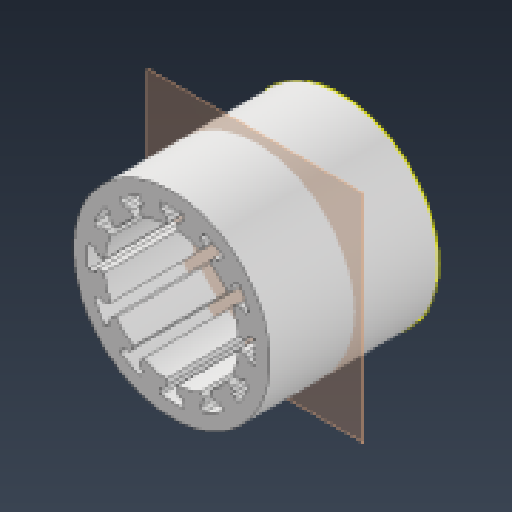
# Autodesk Inventor part: СИСЬКА
Saved by Autodesk Inventor 2026 (Build 300175000, 175)
## iProperties
Created: 2025-10-03
Part Number: СИСЬКА
Material: Типовые
Document SubType Name: Modeling
Designer: Phantom
Density: 1 g/cm^3
Appearance: По умолчанию
Author: Phantom
Autodesk Inventor part; units mm, degrees
ref_plane "YZ Plane" through (0, 0, 0) normal (1, 0, 0) x (0, 1, 0)
ref_plane "XZ Plane" through (0, 0, 0) normal (0, 1, 0) x (-1, 0, 0)
ref_plane "XY Plane" through (0, 0, 0) normal (0, 0, 1) x (1, 0, 0)
sketch "Эскиз1" plane through (0, 0, 0) normal (0, 0, 1) x (1, 0, 0)
  line L0 (-8.756, -8.6711) -> (-8.756, 8.8289)
  line L1 (-8.756, 8.8289) -> (8.744, 8.8289)
  line L2 (8.744, 8.8289) -> (8.744, -8.6711)
  line L3 (8.744, -8.6711) -> (-8.756, -8.6711)
  arc A0 (13.9306, 22.0467) -> (13.3924, 24.6651) centre (12.555, 23.1285) ccw
  line L4 (9.474, 16.3796) -> (13.9306, 22.0467)
  arc A1 (7.3589, 15.8753) -> (9.474, 16.3796) centre (8.0984, 17.4614) ccw
  arc A2 (7.3589, 15.8753) -> (5.5646, 16.5937) centre (-0.006, 0.0789) ccw
  arc A3 (4.3818, 18.4182) -> (5.5646, 16.5937) centre (6.1239, 18.2519) ccw
  line L5 (5.0671, 25.5951) -> (4.3818, 18.4182)
  arc A4 (7.2635, 27.1187) -> (5.0671, 25.5951) centre (6.8092, 25.4288) ccw
  arc A5 (7.2635, 27.1187) -> (-2.0268, 28.0059) centre (-0.006, 0.0789) ccw
  arc A6 (-0.1585, 26.0941) -> (-2.0268, 28.0059) centre (-1.9005, 26.2604) ccw
  line L6 (-0.8438, 18.9172) -> (-0.1585, 26.0941)
  arc A7 (-2.3505, 17.3495) -> (-0.8438, 18.9172) centre (-2.5859, 19.0836) ccw
  arc A8 (-2.3505, 17.3495) -> (-4.2483, 16.9837) centre (-0.006, 0.0789) ccw
  arc A9 (-6.2297, 17.8792) -> (-4.2483, 16.9837) centre (-4.6743, 18.6811) ccw
  line L7 (-9.5333, 24.2872) -> (-6.2297, 17.8792)
  arc A10 (-8.5093, 26.7565) -> (-9.5333, 24.2872) centre (-7.9779, 25.0891) ccw
  arc A11 (-8.5093, 26.7565) -> (-16.8045, 22.48) centre (-0.006, 0.0789) ccw
  arc A12 (-14.1991, 21.8818) -> (-16.8045, 22.48) centre (-15.7546, 21.0799) ccw
  line L8 (-10.8956, 15.4738) -> (-14.1991, 21.8818)
  arc A13 (-11.3155, 13.3403) -> (-10.8956, 15.4738) centre (-12.451, 14.6719) ccw
  arc A14 (-11.3155, 13.3403) -> (-12.7143, 12.0065) centre (-0.006, 0.0789) ccw
  arc A15 (-14.8653, 11.6886) -> (-12.7143, 12.0065) centre (-13.9903, 13.2042) ccw
  line L9 (-21.1089, 15.2934) -> (-14.8653, 11.6886)
  arc A16 (-21.5824, 17.9243) -> (-21.1089, 15.2934) centre (-20.2339, 16.8089) ccw
  arc A17 (-21.5824, 17.9243) -> (-26.2488, 9.842) centre (-0.006, 0.0789) ccw
  arc A18 (-23.7336, 10.7473) -> (-26.2488, 9.842) centre (-24.6086, 9.2318) ccw
  line L10 (-17.49, 7.1425) -> (-23.7336, 10.7473)
  arc A19 (-16.6898, 5.1208) -> (-17.49, 7.1425) centre (-18.365, 5.627) ccw
  arc A20 (-16.6898, 5.1208) -> (-17.1455, 3.2424) centre (-0.006, 0.0789) ccw
  arc A21 (-18.7831, 1.8121) -> (-17.1455, 3.2424) centre (-18.8664, 3.5601) ccw
  line L11 (-25.9845, 1.469) -> (-18.7831, 1.8121)
  arc A22 (-27.8052, 3.4263) -> (-25.9845, 1.469) centre (-26.0677, 3.217) ccw
  arc A23 (-27.8052, 3.4263) -> (-27.3611, -5.8958) centre (-0.006, 0.0789) ccw
  arc A24 (-25.7347, -3.7744) -> (-27.3611, -5.8958) centre (-25.6514, -5.5224) ccw
  line L12 (-18.5334, -3.4313) -> (-25.7347, -3.7744)
  arc A25 (-16.7671, -4.6996) -> (-18.5334, -3.4313) centre (-18.4501, -5.1793) ccw
  arc A26 (-16.7671, -4.6996) -> (-16.135, -6.5261) centre (-0.006, 0.0789) ccw
  arc A27 (-16.7394, -8.6147) -> (-16.135, -6.5261) centre (-17.7545, -7.1892) ccw
  line L13 (-22.6121, -12.7967) -> (-16.7394, -8.6147)
  arc A28 (-25.2019, -12.1345) -> (-22.6121, -12.7967) centre (-23.6272, -11.3712) ccw
  arc A29 (-25.2019, -12.1345) -> (-19.7884, -19.7366) centre (-0.006, 0.0789) ccw
  arc A30 (-19.5671, -17.0727) -> (-19.7884, -19.7366) centre (-18.552, -18.4982) ccw
  line L14 (-13.6944, -12.8907) -> (-19.5671, -17.0727)
  arc A31 (-11.523, -13.0028) -> (-13.6944, -12.8907) centre (-12.6793, -14.3162) ccw
  arc A32 (-11.523, -13.0028) -> (-10.0037, -14.1975) centre (-0.006, 0.0789) ccw
  arc A33 (-9.3829, -16.2814) -> (-10.0037, -14.1975) centre (-11.0075, -15.631) ccw
  line L15 (-12.0624, -22.9745) -> (-9.3829, -16.2814)
  arc A34 (-14.5991, -23.8176) -> (-12.0624, -22.9745) centre (-13.687, -22.3241) ccw
  arc A35 (-14.5991, -23.8176) -> (-5.935, -27.2862) centre (-0.006, 0.0789) ccw
  arc A36 (-7.189, -24.9255) -> (-5.935, -27.2862) centre (-5.5644, -25.5759) ccw
  line L16 (-4.5095, -18.2324) -> (-7.189, -24.9255)
  arc A37 (-2.6222, -17.1526) -> (-4.5095, -18.2324) centre (-2.8849, -18.8828) ccw
  arc A38 (-2.6222, -17.1526) -> (-0.6982, -17.3363) centre (-0.006, 0.0789) ccw
  arc A39 (0.9507, -18.7538) -> (-0.6982, -17.3363) centre (-0.7677, -19.085) ccw
  line L17 (2.3151, -25.833) -> (0.9507, -18.7538)
  arc A40 (0.6369, -27.9137) -> (2.3151, -25.833) centre (0.5967, -26.1642) ccw
  arc A41 (0.6369, -27.9137) -> (9.8009, -26.1475) centre (-0.006, 0.0789) ccw
  arc A42 (7.4696, -24.8396) -> (9.8009, -26.1475) centre (9.188, -24.5084) ccw
  line L18 (6.1065, -17.7672) -> (7.4696, -24.8396)
  arc A43 (7.1038, -15.8414) -> (6.1065, -17.7672) centre (7.8249, -17.436) ccw
  arc A44 (7.1038, -15.8414) -> (8.8253, -14.9478) centre (-0.2779, 0.4827) ccw
  arc A45 (10.981, -15.2474) -> (8.8253, -14.9478) centre (9.7145, -16.455) ccw
  line L19 (15.9557, -20.4647) -> (10.981, -15.2474)
  arc A46 (15.6688, -23.1224) -> (15.9557, -20.4647) centre (14.6891, -21.6723) ccw
  arc A47 (15.6688, -23.1224) -> (22.4232, -16.6821) centre (-0.006, 0.0789) ccw
  arc A48 (19.7548, -16.8422) -> (22.4232, -16.6821) centre (21.0213, -15.6346) ccw
  line L20 (14.7797, -11.6244) -> (19.7548, -16.8422)
  arc A49 (14.5815, -9.4591) -> (14.7797, -11.6244) centre (16.0462, -10.4168) ccw
  arc A50 (14.5815, -9.4591) -> (15.5479, -7.7853) centre (-0.006, 0.0789) ccw
  arc A51 (17.5222, -6.8742) -> (15.5479, -7.7853) centre (17.1096, -8.5749) ccw
  line L21 (24.5285, -8.5739) -> (17.5222, -6.8742)
  arc A52 (25.7241, -10.9648) -> (24.5285, -8.5739) centre (24.1159, -10.2746) ccw
  arc A53 (25.7241, -10.9648) -> (27.9243, -1.8953) centre (-0.006, 0.0789) ccw
  arc A54 (25.7661, -3.4725) -> (27.9243, -1.8953) centre (26.1787, -1.7719) ccw
  line L22 (18.7598, -1.7728) -> (25.7661, -3.4725)
  arc A55 (17.4224, -0.0584) -> (18.7598, -1.7728) centre (19.1724, -0.0722) ccw
  arc A56 (17.4224, -0.0584) -> (17.3305, 1.8722) centre (-0.006, 0.0789) ccw
  arc A57 (18.4988, 3.706) -> (17.3305, 1.8722) centre (19.0712, 2.0523) ccw
  line L23 (25.3118, 6.064) -> (18.4988, 3.706)
  arc A58 (27.6102, 4.699) -> (25.3118, 6.064) centre (25.8842, 4.4103) ccw
  arc A59 (27.6102, 4.699) -> (20.3109, 19.3461) centre (-0.006, 0.0789) ccw
  arc A60 (23.5777, 11.1838) -> (24.694, 13.2663) centre (22.998, 12.835) ccw
  line L24 (16.7752, 8.7957) -> (23.5777, 11.1838)
  arc A61 (14.7201, 9.5059) -> (16.7752, 8.7957) centre (16.1955, 10.4469) ccw
  arc A62 (14.7201, 9.5059) -> (13.592, 11.0753) centre (0.0255, 0.1337) ccw
  arc A63 (13.5738, 13.2496) -> (13.592, 11.0753) centre (14.9541, 12.1739) ccw
  line L25 (18.0053, 18.9363) -> (13.5738, 13.2496)
  arc A64 (20.3109, 19.3461) -> (18.0053, 18.9363) centre (19.3856, 17.8607) ccw
  arc A65 (20.3109, 19.3461) -> (13.3924, 24.6651) centre (-0.006, 0.0789) ccw
  arc A66 (7.3589, 15.8753) -> (5.5646, 16.5937) centre (-0.006, 0.0789) ccw
  arc A67 (7.3589, 15.8753) -> (9.474, 16.3796) centre (8.0984, 17.4614) ccw
  line L26 (9.474, 16.3796) -> (13.9306, 22.0467)
  arc A68 (13.9306, 22.0467) -> (13.3924, 24.6651) centre (12.555, 23.1285) ccw
  arc A69 (13.3924, 24.6651) -> (7.2635, 27.1187) centre (-0.006, 0.0789) ccw
  arc A70 (7.2635, 27.1187) -> (5.0671, 25.5951) centre (6.8092, 25.4288) ccw
  line L27 (5.0671, 25.5951) -> (4.3818, 18.4182)
  arc A71 (4.3818, 18.4182) -> (5.5646, 16.5937) centre (6.1239, 18.2519) ccw
  line L28 (-0.8438, 18.9172) -> (-0.1585, 26.0941)
  arc A72 (-0.1585, 26.0941) -> (-2.0268, 28.0059) centre (-1.9005, 26.2604) ccw
  arc A73 (-2.0268, 28.0059) -> (-8.5093, 26.7565) centre (-0.006, 0.0789) ccw
  arc A74 (-8.5093, 26.7565) -> (-9.5333, 24.2872) centre (-7.9779, 25.0891) ccw
  line L29 (-9.5333, 24.2872) -> (-6.2297, 17.8792)
  arc A75 (-6.2297, 17.8792) -> (-4.2483, 16.9837) centre (-4.6743, 18.6811) ccw
  arc A76 (-2.3505, 17.3495) -> (-4.2483, 16.9837) centre (-0.006, 0.0789) ccw
  arc A77 (-2.3505, 17.3495) -> (-0.8438, 18.9172) centre (-2.5859, 19.0836) ccw
  arc A78 (-11.3155, 13.3403) -> (-12.7143, 12.0065) centre (-0.006, 0.0789) ccw
  arc A79 (-11.3155, 13.3403) -> (-10.8956, 15.4738) centre (-12.451, 14.6719) ccw
  line L30 (-10.8956, 15.4738) -> (-14.1991, 21.8818)
  arc A80 (-14.1991, 21.8818) -> (-16.8045, 22.48) centre (-15.7546, 21.0799) ccw
  arc A81 (-16.8045, 22.48) -> (-21.5824, 17.9243) centre (-0.006, 0.0789) ccw
  arc A82 (-21.5824, 17.9243) -> (-21.1089, 15.2934) centre (-20.2339, 16.8089) ccw
  line L31 (-21.1089, 15.2934) -> (-14.8653, 11.6886)
  arc A83 (-14.8653, 11.6886) -> (-12.7143, 12.0065) centre (-13.9903, 13.2042) ccw
  arc A84 (-26.2488, 9.842) -> (-27.8052, 3.4263) centre (-0.006, 0.0789) ccw
  arc A85 (-27.8052, 3.4263) -> (-25.9845, 1.469) centre (-26.0677, 3.217) ccw
  line L32 (-25.9845, 1.469) -> (-18.7831, 1.8121)
  arc A86 (-18.7831, 1.8121) -> (-17.1455, 3.2424) centre (-18.8664, 3.5601) ccw
  arc A87 (-16.6898, 5.1208) -> (-17.1455, 3.2424) centre (-0.006, 0.0789) ccw
  arc A88 (-16.6898, 5.1208) -> (-17.49, 7.1425) centre (-18.365, 5.627) ccw
  line L33 (-17.49, 7.1425) -> (-23.7336, 10.7473)
  arc A89 (-23.7336, 10.7473) -> (-26.2488, 9.842) centre (-24.6086, 9.2318) ccw
  arc A90 (-27.3611, -5.8958) -> (-25.2019, -12.1345) centre (-0.006, 0.0789) ccw
  arc A91 (-25.2019, -12.1345) -> (-22.6121, -12.7967) centre (-23.6272, -11.3712) ccw
  line L34 (-22.6121, -12.7967) -> (-16.7394, -8.6147)
  arc A92 (-16.7394, -8.6147) -> (-16.135, -6.5261) centre (-17.7545, -7.1892) ccw
  arc A93 (-16.7671, -4.6996) -> (-16.135, -6.5261) centre (-0.006, 0.0789) ccw
  arc A94 (-16.7671, -4.6996) -> (-18.5334, -3.4313) centre (-18.4501, -5.1793) ccw
  line L35 (-18.5334, -3.4313) -> (-25.7347, -3.7744)
  arc A95 (-25.7347, -3.7744) -> (-27.3611, -5.8958) centre (-25.6514, -5.5224) ccw
  arc A96 (-5.935, -27.2862) -> (0.6369, -27.9137) centre (-0.006, 0.0789) ccw
  arc A97 (0.6369, -27.9137) -> (2.3151, -25.833) centre (0.5967, -26.1642) ccw
  line L36 (2.3151, -25.833) -> (0.9507, -18.7538)
  arc A98 (0.9507, -18.7538) -> (-0.6982, -17.3363) centre (-0.7677, -19.085) ccw
  arc A99 (-2.6222, -17.1526) -> (-0.6982, -17.3363) centre (-0.006, 0.0789) ccw
  arc A100 (-2.6222, -17.1526) -> (-4.5095, -18.2324) centre (-2.8849, -18.8828) ccw
  line L37 (-4.5095, -18.2324) -> (-7.189, -24.9255)
  arc A101 (-7.189, -24.9255) -> (-5.935, -27.2862) centre (-5.5644, -25.5759) ccw
  arc A102 (9.8009, -26.1475) -> (15.6688, -23.1224) centre (-0.006, 0.0789) ccw
  arc A103 (15.6688, -23.1224) -> (15.9557, -20.4647) centre (14.6891, -21.6723) ccw
  line L38 (15.9557, -20.4647) -> (10.981, -15.2474)
  arc A104 (10.981, -15.2474) -> (8.8253, -14.9478) centre (9.7145, -16.455) ccw
  arc A105 (7.1038, -15.8414) -> (8.8253, -14.9478) centre (-0.2779, 0.4827) ccw
  arc A106 (7.1038, -15.8414) -> (6.1065, -17.7672) centre (7.8249, -17.436) ccw
  line L39 (6.1065, -17.7672) -> (7.4696, -24.8396)
  arc A107 (7.4696, -24.8396) -> (9.8009, -26.1475) centre (9.188, -24.5084) ccw
  arc A108 (-19.7884, -19.7366) -> (-14.5991, -23.8176) centre (-0.006, 0.0789) ccw
  arc A109 (-14.5991, -23.8176) -> (-12.0624, -22.9745) centre (-13.687, -22.3241) ccw
  line L40 (-12.0624, -22.9745) -> (-9.3829, -16.2814)
  arc A110 (-9.3829, -16.2814) -> (-10.0037, -14.1975) centre (-11.0075, -15.631) ccw
  arc A111 (-11.523, -13.0028) -> (-10.0037, -14.1975) centre (-0.006, 0.0789) ccw
  arc A112 (-11.523, -13.0028) -> (-13.6944, -12.8907) centre (-12.6793, -14.3162) ccw
  line L41 (-13.6944, -12.8907) -> (-19.5671, -17.0727)
  arc A113 (-19.5671, -17.0727) -> (-19.7884, -19.7366) centre (-18.552, -18.4982) ccw
  arc A114 (14.5815, -9.4591) -> (15.5479, -7.7853) centre (-0.006, 0.0789) ccw
  arc A115 (14.5815, -9.4591) -> (14.7797, -11.6244) centre (16.0462, -10.4168) ccw
  line L42 (14.7797, -11.6244) -> (19.7548, -16.8422)
  arc A116 (19.7548, -16.8422) -> (22.4232, -16.6821) centre (21.0213, -15.6346) ccw
  arc A117 (22.4232, -16.6821) -> (25.7241, -10.9648) centre (-0.006, 0.0789) ccw
  arc A118 (25.7241, -10.9648) -> (24.5285, -8.5739) centre (24.1159, -10.2746) ccw
  line L43 (24.5285, -8.5739) -> (17.5222, -6.8742)
  arc A119 (17.5222, -6.8742) -> (15.5479, -7.7853) centre (17.1096, -8.5749) ccw
  line L44 (18.7598, -1.7728) -> (25.7661, -3.4725)
  arc A120 (25.7661, -3.4725) -> (27.9243, -1.8953) centre (26.1787, -1.7719) ccw
  arc A121 (27.9243, -1.8953) -> (27.6102, 4.699) centre (-0.006, 0.0789) ccw
  arc A122 (27.6102, 4.699) -> (25.3118, 6.064) centre (25.8842, 4.4103) ccw
  line L45 (25.3118, 6.064) -> (18.4988, 3.706)
  arc A123 (18.4988, 3.706) -> (17.3305, 1.8722) centre (19.0712, 2.0523) ccw
  arc A124 (17.4224, -0.0584) -> (17.3305, 1.8722) centre (-0.006, 0.0789) ccw
  arc A125 (17.4224, -0.0584) -> (18.7598, -1.7728) centre (19.1724, -0.0722) ccw
  circle A126 centre (-0.006, 0.0789) radius 35
  point P0 (0, 0)
  point P1 (-1.0694, -0.3768)
  point P2 (13.3924, 24.6651)
  point P3 (4.3818, 18.4182)
  point P4 (-2.0268, 28.0059)
  point P5 (-4.2483, 16.9837)
  point P6 (-6.2297, 17.8792)
  point P7 (-8.5093, 26.7565)
  point P8 (-14.8653, 11.6886)
  point P9 (-27.8052, 3.4263)
  point P10 (-27.3611, -5.8958)
  point P11 (-25.2019, -12.1345)
  point P12 (-5.935, -27.2862)
  point P13 (0.6369, -27.9137)
  point P14 (9.8009, -26.1475)
  point P15 (15.6688, -23.1224)
  point P16 (18.7598, -1.7728)
  dimension "d0" = 70
  constraints: 253 point on circle, 127 centre point, 92 end point, 1 coincident
  measures "d0" diameter of A126
extrude "Выдавливание1" add sketch "Эскиз1" along normal blind 60 contours L4 A1 A2 A3 L5 A4 A69 A0 | A0 A65 A64 L25 A63 A62 A61 L24 A60 A59 A58 L23 A57 A56 A55 L22 A54 A53 A52 L21 A51 A50 A49 L20 A48 A47 A46 L19 A45 A44 A43 L18 A42 A41 A40 L17 A39 A38 A37 L16 A36 A35 A34 L15 A33 A32 A31 L14 A30 A29 A28 L13 A27 A26 A25 L12 A24 A23 A22 L11 A21 A20 A19 L10 A18 A17 A16 L9 A15 A14 A13 L8 A12 A11 A10 L7 A9 A8 A7 L6 A6 A5 A4 L5 A3 A2 A1 L4 | A59 A60 L24 A61 A62 A63 L25 A64 | A6 L6 A7 A8 A9 L7 A10 A73 | A121 A54 L22 A55 A56 A57 L23 A58 | A12 L8 A13 A14 A15 L9 A16 A81 | A117 A48 L20 A49 A50 A51 L21 A52 | A18 L10 A19 A20 A21 L11 A22 A84 | A102 A42 L18 A43 A44 A45 L19 A46 | A24 L12 A25 A26 A27 L13 A28 A90 | A96 A36 L16 A37 A38 A39 L17 A40 | A30 L14 A31 A32 A33 L15 A34 A108 | A126
sketch "Эскиз4" plane through (-0.006, 0.0789, 60) normal (0, 0, 1) x (1, 0, 0)
  circle A0 centre (0, 0) radius 35 projected
  circle A1 centre (0, 0) radius 30
  line L0 (0, 30) -> (0, -30)
  line L1 (-4, 30) -> (-4, 28)
  line L2 (4, 30) -> (4, 28)
  line L3 (3, 27) -> (3, 27)
  line L4 (-2, 26) -> (-2, -30)
  line L5 (2, 26) -> (2, -30)
  arc A2 (-2, 26) -> (-3, 27) centre (-3, 26) ccw
  arc A3 (-4, 28) -> (-3, 27) centre (-3, 28) ccw
  arc A4 (3, 27) -> (4, 28) centre (3, 28) ccw
  arc A5 (3, 27) -> (2, 26) centre (3, 26) ccw
  line L6 (-4, 34.038) -> (4, 34.038)
  circle A6 centre (0, 0) radius 24
  line L7 (-18.4641, 23.9808) -> (-17.4641, 22.2487)
  arc A7 (-17.4641, 22.2487) -> (-16.0981, 21.8827) centre (-16.5981, 22.7487) ccw
  arc A8 (-14.7321, 21.5167) -> (-16.0981, 21.8827) centre (-15.5981, 21.0167) ccw
  line L8 (-14.7321, 21.5167) -> (13.2679, -26.9808)
  line L9 (-11.2679, 23.5167) -> (16.7321, -24.9808)
  arc A9 (-10.9019, 24.8827) -> (-11.2679, 23.5167) centre (-10.4019, 24.0167) ccw
  arc A10 (-10.9019, 24.8827) -> (-10.5359, 26.2487) centre (-11.4019, 25.7487) ccw
  line L10 (-11.5359, 27.9808) -> (-10.5359, 26.2487)
  line L11 (-27.9808, 11.5359) -> (-26.2487, 10.5359)
  arc A11 (-26.2487, 10.5359) -> (-24.8827, 10.9019) centre (-25.7487, 11.4019) ccw
  arc A12 (-23.5167, 11.2679) -> (-24.8827, 10.9019) centre (-24.0167, 10.4019) ccw
  line L12 (-23.5167, 11.2679) -> (24.9808, -16.7321)
  line L13 (-21.5167, 14.7321) -> (26.9808, -13.2679)
  arc A13 (-21.8827, 16.0981) -> (-21.5167, 14.7321) centre (-21.0167, 15.5981) ccw
  arc A14 (-21.8827, 16.0981) -> (-22.2487, 17.4641) centre (-22.7487, 16.5981) ccw
  line L14 (-23.9808, 18.4641) -> (-22.2487, 17.4641)
  line L15 (-30, -4) -> (-28, -4)
  arc A15 (-28, -4) -> (-27, -3) centre (-28, -3) ccw
  arc A16 (-26, -2) -> (-27, -3) centre (-26, -3) ccw
  line L16 (-26, -2) -> (30, -2)
  line L17 (-26, 2) -> (30, 2)
  arc A17 (-27, 3) -> (-26, 2) centre (-26, 3) ccw
  arc A18 (-27, 3) -> (-28, 4) centre (-28, 3) ccw
  line L18 (-30, 4) -> (-28, 4)
  line L19 (-23.9808, -18.4641) -> (-22.2487, -17.4641)
  arc A19 (-22.2487, -17.4641) -> (-21.8827, -16.0981) centre (-22.7487, -16.5981) ccw
  arc A20 (-21.5167, -14.7321) -> (-21.8827, -16.0981) centre (-21.0167, -15.5981) ccw
  line L20 (-21.5167, -14.7321) -> (26.9808, 13.2679)
  line L21 (-23.5167, -11.2679) -> (24.9808, 16.7321)
  arc A21 (-24.8827, -10.9019) -> (-23.5167, -11.2679) centre (-24.0167, -10.4019) ccw
  arc A22 (-24.8827, -10.9019) -> (-26.2487, -10.5359) centre (-25.7487, -11.4019) ccw
  line L22 (-27.9808, -11.5359) -> (-26.2487, -10.5359)
  line L23 (-11.5359, -27.9808) -> (-10.5359, -26.2487)
  arc A23 (-10.5359, -26.2487) -> (-10.9019, -24.8827) centre (-11.4019, -25.7487) ccw
  arc A24 (-11.2679, -23.5167) -> (-10.9019, -24.8827) centre (-10.4019, -24.0167) ccw
  line L24 (-11.2679, -23.5167) -> (16.7321, 24.9808)
  line L25 (-14.7321, -21.5167) -> (13.2679, 26.9808)
  arc A25 (-16.0981, -21.8827) -> (-14.7321, -21.5167) centre (-15.5981, -21.0167) ccw
  arc A26 (-16.0981, -21.8827) -> (-17.4641, -22.2487) centre (-16.5981, -22.7487) ccw
  line L26 (-18.4641, -23.9808) -> (-17.4641, -22.2487)
  line L27 (4, -30) -> (4, -28)
  arc A27 (4, -28) -> (3, -27) centre (3, -28) ccw
  arc A28 (2, -26) -> (3, -27) centre (3, -26) ccw
  line L28 (2, -26) -> (2, 30)
  line L29 (-2, -26) -> (-2, 30)
  arc A29 (-3, -27) -> (-2, -26) centre (-3, -26) ccw
  arc A30 (-3, -27) -> (-4, -28) centre (-3, -28) ccw
  line L30 (-4, -30) -> (-4, -28)
  line L31 (18.4641, -23.9808) -> (17.4641, -22.2487)
  arc A31 (17.4641, -22.2487) -> (16.0981, -21.8827) centre (16.5981, -22.7487) ccw
  arc A32 (14.7321, -21.5167) -> (16.0981, -21.8827) centre (15.5981, -21.0167) ccw
  line L32 (14.7321, -21.5167) -> (-13.2679, 26.9808)
  line L33 (11.2679, -23.5167) -> (-16.7321, 24.9808)
  arc A33 (10.9019, -24.8827) -> (11.2679, -23.5167) centre (10.4019, -24.0167) ccw
  arc A34 (10.9019, -24.8827) -> (10.5359, -26.2487) centre (11.4019, -25.7487) ccw
  line L34 (11.5359, -27.9808) -> (10.5359, -26.2487)
  line L35 (27.9808, -11.5359) -> (26.2487, -10.5359)
  arc A35 (26.2487, -10.5359) -> (24.8827, -10.9019) centre (25.7487, -11.4019) ccw
  arc A36 (23.5167, -11.2679) -> (24.8827, -10.9019) centre (24.0167, -10.4019) ccw
  line L36 (23.5167, -11.2679) -> (-24.9808, 16.7321)
  line L37 (21.5167, -14.7321) -> (-26.9808, 13.2679)
  arc A37 (21.8827, -16.0981) -> (21.5167, -14.7321) centre (21.0167, -15.5981) ccw
  arc A38 (21.8827, -16.0981) -> (22.2487, -17.4641) centre (22.7487, -16.5981) ccw
  line L38 (23.9808, -18.4641) -> (22.2487, -17.4641)
  line L39 (30, 4) -> (28, 4)
  arc A39 (28, 4) -> (27, 3) centre (28, 3) ccw
  arc A40 (26, 2) -> (27, 3) centre (26, 3) ccw
  line L40 (26, 2) -> (-30, 2)
  line L41 (26, -2) -> (-30, -2)
  arc A41 (27, -3) -> (26, -2) centre (26, -3) ccw
  arc A42 (27, -3) -> (28, -4) centre (28, -3) ccw
  line L42 (30, -4) -> (28, -4)
  line L43 (23.9808, 18.4641) -> (22.2487, 17.4641)
  arc A43 (22.2487, 17.4641) -> (21.8827, 16.0981) centre (22.7487, 16.5981) ccw
  arc A44 (21.5167, 14.7321) -> (21.8827, 16.0981) centre (21.0167, 15.5981) ccw
  line L44 (21.5167, 14.7321) -> (-26.9808, -13.2679)
  line L45 (23.5167, 11.2679) -> (-24.9808, -16.7321)
  arc A45 (24.8827, 10.9019) -> (23.5167, 11.2679) centre (24.0167, 10.4019) ccw
  arc A46 (24.8827, 10.9019) -> (26.2487, 10.5359) centre (25.7487, 11.4019) ccw
  line L46 (27.9808, 11.5359) -> (26.2487, 10.5359)
  line L47 (11.5359, 27.9808) -> (10.5359, 26.2487)
  arc A47 (10.5359, 26.2487) -> (10.9019, 24.8827) centre (11.4019, 25.7487) ccw
  arc A48 (11.2679, 23.5167) -> (10.9019, 24.8827) centre (10.4019, 24.0167) ccw
  line L48 (11.2679, 23.5167) -> (-16.7321, -24.9808)
  line L49 (14.7321, 21.5167) -> (-13.2679, -26.9808)
  arc A49 (16.0981, 21.8827) -> (14.7321, 21.5167) centre (15.5981, 21.0167) ccw
  arc A50 (16.0981, 21.8827) -> (17.4641, 22.2487) centre (16.5981, 22.7487) ccw
  line L50 (18.4641, 23.9808) -> (17.4641, 22.2487)
  point P0 (-20.4831, 27.4778)
  point P1 (-31.4778, 13.5549)
  point P2 (-34.038, -4)
  point P3 (-27.4778, -20.4831)
  point P4 (-13.5549, -31.4778)
  point P5 (4, -34.038)
  point P6 (20.4831, -27.4778)
  point P7 (31.4778, -13.5549)
  point P8 (34.038, 4)
  point P9 (27.4778, 20.4831)
  point P10 (13.5549, 31.4778)
  point P11 (-13.6903, 19.7123)
  point P12 (-10.2262, 21.7123)
  point P13 (-10.9019, 24.8827)
  point P14 (-11.402, 27.7488)
  point P15 (-18.3302, 23.7488)
  point P16 (4, 29.7321)
  point P17 (-4, 29.7321)
  point P18 (-2, 23.9165)
  point P19 (2, 23.9165)
  point P20 (16.0981, 21.8827)
  point P21 (18.3302, 23.7488)
  point P22 (11.402, 27.7488)
  point P23 (10.2262, 21.7123)
  point P24 (13.6903, 19.7123)
  point P25 (21.5167, 14.7321)
  point P26 (19.7123, 13.6903)
  point P27 (21.7123, 10.2262)
  point P28 (24.8827, 10.9019)
  point P29 (27.7488, 11.402)
  point P30 (23.7488, 18.3302)
  point P31 (23.9165, 2)
  point P32 (23.9165, -2)
  point P33 (29.7321, -4)
  point P34 (29.7321, 4)
  point P35 (23.7488, -18.3302)
  point P36 (27.7488, -11.402)
  point P37 (23.5167, -11.2679)
  point P38 (21.7123, -10.2262)
  point P39 (19.7123, -13.6903)
  point P40 (10.9019, -24.8827)
  point P41 (11.402, -27.7488)
  point P42 (18.3302, -23.7488)
  point P43 (13.6903, -19.7123)
  point P44 (10.2262, -21.7123)
  point P45 (-2, -23.9165)
  point P46 (-4, -29.7321)
  point P47 (4, -29.7321)
  point P48 (2, -23.9165)
  point P49 (-10.2262, -21.7123)
  point P50 (-13.6903, -19.7123)
  point P51 (-18.3302, -23.7488)
  point P52 (-11.402, -27.7488)
  point P53 (-19.7123, -13.6903)
  point P54 (-21.7123, -10.2262)
  point P55 (-24.8827, -10.9019)
  point P56 (-27.7488, -11.402)
  point P57 (-23.7488, -18.3302)
  point P58 (-23.9165, -2)
  point P59 (-23.9165, 2)
  point P60 (-29.7321, 4)
  point P61 (-29.7321, -4)
  point P62 (-21.7123, 10.2262)
  point P63 (-19.7123, 13.6903)
  point P64 (-23.7488, 18.3302)
  point P65 (-27.7488, 11.402)
  dimension "d7" = 60
  dimension "d15" = 48
  dimension "d8" = 4
  dimension "d9" = 4
  dimension "d10" = 3
  dimension "d11" = 2
  dimension "d12" = 2
  dimension "d13" = 1
  dimension "d14" = 1
  dimension "d18" = 360
  constraints: 102 end point, 96 point on circle, 48 centre point, 12 point on line, 8 tangent, 4 parallel, 2 coincident, 2 equal radius, 2 horizontal, 1 vertical, 295 other
  measures "d8" distance between parallel lines of L0 L1
  measures "d9" distance between parallel lines of L0 L2
  measures "d10" distance from line of L0.start L3
  measures "d11" distance between parallel lines of L0 L4
  measures "d12" distance between parallel lines of L0 L5
  measures "d13" radius of A2
  measures "d14" radius of A4
extrude "Выдавливание3" cut sketch "Эскиз4" against normal blind 60 contours A1 L16 A6 L17 | L17 A40 A39 L39 A1 | A1 L42 A42 A41 L16 | L46 A46 A45 L20 A1 | L17 L20 A6 | A6 L16 L13 L20 L17 | A1 L13 A36 A35 L35 | A6 L13 L16 | L20 A6 L21 A1 | L20 L17 L24 L21 A6 | L20 L13 L24 L17 | A1 L12 A6 L13 | A6 L12 L9 L16 L13 | L16 L9 L20 L13 | L21 A44 A43 L43 A1 | L21 L24 A6 | L24 L13 L5 L17 | L17 L5 L21 L24 | L20 L9 L24 L13 | A1 L38 A38 A37 L12 | A6 L9 L12 | L16 L5 L20 L9 | L9 L12 L5 L16 | L24 L21 L5 L25 A6 | A6 L25 A1 L24 | L17 L9 L21 L5 | L5 L13 L9 L17 | L24 L9 L5 L13 | L20 L5 L24 L9 | L9 A1 L8 A6 | A6 L8 L5 L12 L9 | L16 L24 L20 L5 | L5 L12 L24 L16 | L50 A50 A49 L24 A1 | L25 L5 A6 | L21 L9 L25 L5 | L5 L9 L13 | L17 L13 L21 L9 | L9 L13 L17 | L24 L5 L9 | L20 L24 L5 | A1 L9 A32 A31 L31 | A6 L5 L8 | L5 L8 L24 L12 | L24 L12 L20 L16 | L16 L20 L24 | A6 L0 A1 L28 L5 | L5 L25 L0 A6 | A48 A47 L47 A1 L25 | L21 L0 L9 | L5 L24 L20 L16 L0 L17 L13 L9 | L17 L0 L13 | A6 L0 L8 L5 | L5 A1 L0 A6 | L8 A1 L34 A34 A33 | L24 L0 L12 | L20 L0 L16 | L28 A1 L2 A4 A5 | A6 L4 L29 A1 L0 | L0 L9 L4 A6 | L25 L13 L4 L9 | L0 L13 L25 | L21 L17 L25 L13 | L0 L17 L21 | L0 L16 L12 L8 L4 L25 L21 L17 | A28 A27 L27 A1 L5 | A6 L4 L24 L0 | L0 A1 L4 A6 | L8 L20 L0 | L24 L4 L20 L8 | L12 L16 L0 | L20 L8 L16 L12 | L4 L9 A6 | L4 L13 L8 A6 L9 | L25 L17 L4 L13 | L21 L25 L17 | A6 L24 L4 | L20 L4 L16 L8 | L24 A6 L25 L20 L4 | L16 L8 L12 | L29 A2 A3 L1 A1 | A6 L8 L33 A1 L32 L9 | L4 L17 L8 L13 | L25 L21 L4 L17 | L25 L4 L21 | A1 L30 A30 A29 L4 | L24 L49 A1 L48 L25 A6 | L16 L4 L12 L8 | L20 L25 L16 L4 | L12 L4 L8 | L8 L13 A6 | L32 A1 L10 A10 A9 | L4 L21 L8 L17 | L8 L17 L12 A6 L13 | L4 L25 L8 L21 | L4 L8 L25 | A6 L20 L25 | A24 A23 L23 A1 L49 | L16 L25 L12 L4 | L20 A6 L21 L16 L25 | L4 L12 L25 L8 | A6 L12 L37 A1 L36 L13 | A8 A7 L7 A1 L33 | L8 L21 L12 L17 | L8 L25 L12 L21 | L20 L45 A1 L44 L21 A6 | L48 A1 L26 A26 A25 | L16 L21 L12 L25 | L12 L17 A6 | L36 A1 L14 A14 A13 | L12 L21 L16 A6 L17 | A6 L16 L21 | A20 A19 L19 A1 L45 | A6 L16 L41 A1 L40 L17 | A12 A11 L11 A1 L37 | L44 A1 L22 A22 A21 | L40 A1 L18 A18 A17 | A16 A15 L15 A1 L41
sketch "Эскиз5" plane through (-0.006, 0.0789, 0) normal (0, 0, -1) x (-1, 0, 0)
  arc A0 (26, 2) -> (27, 3) centre (26, 3) ccw projected
  arc A1 (28, 4) -> (27, 3) centre (28, 3) ccw projected
  line L0 (28, 4) -> (29.7321, 4) projected
  arc A2 (29.7321, -4) -> (29.7321, 4) centre (0, 0) ccw projected
  line L1 (29.7321, -4) -> (28, -4) projected
  arc A3 (27, -3) -> (28, -4) centre (28, -3) ccw projected
  arc A4 (27, -3) -> (26, -2) centre (26, -3) ccw projected
  line L2 (26, -2) -> (23.9165, -2) projected
  arc A5 (21.7123, -10.2262) -> (23.9165, -2) centre (0, 0) ccw projected
  line L3 (21.7123, -10.2262) -> (23.5167, -11.2679) projected
  arc A6 (23.5167, -11.2679) -> (24.8827, -10.9019) centre (24.0167, -10.4019) ccw projected
  arc A7 (26.2487, -10.5359) -> (24.8827, -10.9019) centre (25.7487, -11.4019) ccw projected
  line L4 (26.2487, -10.5359) -> (27.7488, -11.402) projected
  arc A8 (23.7488, -18.3302) -> (27.7488, -11.402) centre (0, 0) ccw projected
  line L5 (23.7488, -18.3302) -> (22.2487, -17.4641) projected
  arc A9 (21.8827, -16.0981) -> (22.2487, -17.4641) centre (22.7487, -16.5981) ccw projected
  arc A10 (21.8827, -16.0981) -> (21.5167, -14.7321) centre (21.0167, -15.5981) ccw projected
  line L6 (21.5167, -14.7321) -> (19.7123, -13.6903) projected
  arc A11 (13.6903, -19.7123) -> (19.7123, -13.6903) centre (0, 0) ccw projected
  line L7 (13.6903, -19.7123) -> (14.7321, -21.5167) projected
  arc A12 (14.7321, -21.5167) -> (16.0981, -21.8827) centre (15.5981, -21.0167) ccw projected
  arc A13 (17.4641, -22.2487) -> (16.0981, -21.8827) centre (16.5981, -22.7487) ccw projected
  line L8 (17.4641, -22.2487) -> (18.3302, -23.7488) projected
  arc A14 (11.402, -27.7488) -> (18.3302, -23.7488) centre (0, 0) ccw projected
  line L9 (11.402, -27.7488) -> (10.5359, -26.2487) projected
  arc A15 (10.9019, -24.8827) -> (10.5359, -26.2487) centre (11.4019, -25.7487) ccw projected
  arc A16 (10.9019, -24.8827) -> (11.2679, -23.5167) centre (10.4019, -24.0167) ccw projected
  line L10 (11.2679, -23.5167) -> (10.2262, -21.7123) projected
  arc A17 (2, -23.9165) -> (10.2262, -21.7123) centre (0, 0) ccw projected
  line L11 (2, -23.9165) -> (2, -26) projected
  arc A18 (2, -26) -> (3, -27) centre (3, -26) ccw projected
  arc A19 (4, -28) -> (3, -27) centre (3, -28) ccw projected
  line L12 (4, -28) -> (4, -29.7321) projected
  arc A20 (-4, -29.7321) -> (4, -29.7321) centre (0, 0) ccw projected
  line L13 (-4, -29.7321) -> (-4, -28) projected
  arc A21 (-3, -27) -> (-4, -28) centre (-3, -28) ccw projected
  arc A22 (-3, -27) -> (-2, -26) centre (-3, -26) ccw projected
  line L14 (-2, -26) -> (-2, -23.9165) projected
  arc A23 (-10.2262, -21.7123) -> (-2, -23.9165) centre (0, 0) ccw projected
  line L15 (-10.2262, -21.7123) -> (-11.2679, -23.5167) projected
  arc A24 (-11.2679, -23.5167) -> (-10.9019, -24.8827) centre (-10.4019, -24.0167) ccw projected
  arc A25 (-10.5359, -26.2487) -> (-10.9019, -24.8827) centre (-11.4019, -25.7487) ccw projected
  line L16 (-10.5359, -26.2487) -> (-11.402, -27.7488) projected
  arc A26 (-18.3302, -23.7488) -> (-11.402, -27.7488) centre (0, 0) ccw projected
  line L17 (-18.3302, -23.7488) -> (-17.4641, -22.2487) projected
  arc A27 (-16.0981, -21.8827) -> (-17.4641, -22.2487) centre (-16.5981, -22.7487) ccw projected
  arc A28 (-16.0981, -21.8827) -> (-14.7321, -21.5167) centre (-15.5981, -21.0167) ccw projected
  line L18 (-14.7321, -21.5167) -> (-13.6903, -19.7123) projected
  arc A29 (-19.7123, -13.6903) -> (-13.6903, -19.7123) centre (0, 0) ccw projected
  line L19 (-19.7123, -13.6903) -> (-21.5167, -14.7321) projected
  arc A30 (-21.5167, -14.7321) -> (-21.8827, -16.0981) centre (-21.0167, -15.5981) ccw projected
  arc A31 (-22.2487, -17.4641) -> (-21.8827, -16.0981) centre (-22.7487, -16.5981) ccw projected
  line L20 (-22.2487, -17.4641) -> (-23.7488, -18.3302) projected
  arc A32 (-27.7488, -11.402) -> (-23.7488, -18.3302) centre (0, 0) ccw projected
  line L21 (-27.7488, -11.402) -> (-26.2487, -10.5359) projected
  arc A33 (-24.8827, -10.9019) -> (-26.2487, -10.5359) centre (-25.7487, -11.4019) ccw projected
  arc A34 (-24.8827, -10.9019) -> (-23.5167, -11.2679) centre (-24.0167, -10.4019) ccw projected
  line L22 (-23.5167, -11.2679) -> (-21.7123, -10.2262) projected
  arc A35 (-23.9165, -2) -> (-21.7123, -10.2262) centre (0, 0) ccw projected
  line L23 (-23.9165, -2) -> (-26, -2) projected
  arc A36 (-26, -2) -> (-27, -3) centre (-26, -3) ccw projected
  arc A37 (-28, -4) -> (-27, -3) centre (-28, -3) ccw projected
  line L24 (-28, -4) -> (-29.7321, -4) projected
  arc A38 (-29.7321, 4) -> (-29.7321, -4) centre (0, 0) ccw projected
  line L25 (-29.7321, 4) -> (-28, 4) projected
  arc A39 (-27, 3) -> (-28, 4) centre (-28, 3) ccw projected
  arc A40 (-27, 3) -> (-26, 2) centre (-26, 3) ccw projected
  line L26 (-26, 2) -> (-23.9165, 2) projected
  arc A41 (-21.7123, 10.2262) -> (-23.9165, 2) centre (0, 0) ccw projected
  line L27 (-21.7123, 10.2262) -> (-23.5167, 11.2679) projected
  arc A42 (-23.5167, 11.2679) -> (-24.8827, 10.9019) centre (-24.0167, 10.4019) ccw projected
  arc A43 (-26.2487, 10.5359) -> (-24.8827, 10.9019) centre (-25.7487, 11.4019) ccw projected
  line L28 (-26.2487, 10.5359) -> (-27.7488, 11.402) projected
  arc A44 (-23.7488, 18.3302) -> (-27.7488, 11.402) centre (0, 0) ccw projected
  line L29 (-23.7488, 18.3302) -> (-22.2487, 17.4641) projected
  arc A45 (-21.8827, 16.0981) -> (-22.2487, 17.4641) centre (-22.7487, 16.5981) ccw projected
  arc A46 (-21.8827, 16.0981) -> (-21.5167, 14.7321) centre (-21.0167, 15.5981) ccw projected
  line L30 (-21.5167, 14.7321) -> (-19.7123, 13.6903) projected
  arc A47 (-13.6903, 19.7123) -> (-19.7123, 13.6903) centre (0, 0) ccw projected
  line L31 (-13.6903, 19.7123) -> (-14.7321, 21.5167) projected
  arc A48 (-14.7321, 21.5167) -> (-16.0981, 21.8827) centre (-15.5981, 21.0167) ccw projected
  arc A49 (-17.4641, 22.2487) -> (-16.0981, 21.8827) centre (-16.5981, 22.7487) ccw projected
  line L32 (-17.4641, 22.2487) -> (-18.3302, 23.7488) projected
  arc A50 (-11.402, 27.7488) -> (-18.3302, 23.7488) centre (0, 0) ccw projected
  line L33 (-11.402, 27.7488) -> (-10.5359, 26.2487) projected
  arc A51 (-10.9019, 24.8827) -> (-10.5359, 26.2487) centre (-11.4019, 25.7487) ccw projected
  arc A52 (-10.9019, 24.8827) -> (-11.2679, 23.5167) centre (-10.4019, 24.0167) ccw projected
  line L34 (-11.2679, 23.5167) -> (-10.2262, 21.7123) projected
  arc A53 (-2, 23.9165) -> (-10.2262, 21.7123) centre (0, 0) ccw projected
  line L35 (-2, 23.9165) -> (-2, 26) projected
  arc A54 (-2, 26) -> (-3, 27) centre (-3, 26) ccw projected
  arc A55 (-4, 28) -> (-3, 27) centre (-3, 28) ccw projected
  line L36 (-4, 28) -> (-4, 29.7321) projected
  arc A56 (4, 29.7321) -> (-4, 29.7321) centre (0, 0) ccw projected
  line L37 (4, 29.7321) -> (4, 28) projected
  arc A57 (3, 27) -> (4, 28) centre (3, 28) ccw projected
  arc A58 (3, 27) -> (2, 26) centre (3, 26) ccw projected
  line L38 (2, 26) -> (2, 23.9165) projected
  arc A59 (10.2262, 21.7123) -> (2, 23.9165) centre (0, 0) ccw projected
  line L39 (10.2262, 21.7123) -> (11.2679, 23.5167) projected
  arc A60 (11.2679, 23.5167) -> (10.9019, 24.8827) centre (10.4019, 24.0167) ccw projected
  arc A61 (10.5359, 26.2487) -> (10.9019, 24.8827) centre (11.4019, 25.7487) ccw projected
  line L40 (10.5359, 26.2487) -> (11.402, 27.7488) projected
  arc A62 (18.3302, 23.7488) -> (11.402, 27.7488) centre (0, 0) ccw projected
  line L41 (18.3302, 23.7488) -> (17.4641, 22.2487) projected
  arc A63 (16.0981, 21.8827) -> (17.4641, 22.2487) centre (16.5981, 22.7487) ccw projected
  arc A64 (16.0981, 21.8827) -> (14.7321, 21.5167) centre (15.5981, 21.0167) ccw projected
  line L42 (14.7321, 21.5167) -> (13.6903, 19.7123) projected
  arc A65 (19.7123, 13.6903) -> (13.6903, 19.7123) centre (0, 0) ccw projected
  line L43 (19.7123, 13.6903) -> (21.5167, 14.7321) projected
  arc A66 (21.5167, 14.7321) -> (21.8827, 16.0981) centre (21.0167, 15.5981) ccw projected
  arc A67 (22.2487, 17.4641) -> (21.8827, 16.0981) centre (22.7487, 16.5981) ccw projected
  line L44 (22.2487, 17.4641) -> (23.7488, 18.3302) projected
  arc A68 (27.7488, 11.402) -> (23.7488, 18.3302) centre (0, 0) ccw projected
  line L45 (27.7488, 11.402) -> (26.2487, 10.5359) projected
  arc A69 (24.8827, 10.9019) -> (26.2487, 10.5359) centre (25.7487, 11.4019) ccw projected
  arc A70 (24.8827, 10.9019) -> (23.5167, 11.2679) centre (24.0167, 10.4019) ccw projected
  line L46 (23.5167, 11.2679) -> (21.7123, 10.2262) projected
  arc A71 (23.9165, 2) -> (21.7123, 10.2262) centre (0, 0) ccw projected
  line L47 (23.9165, 2) -> (26, 2) projected
  circle A72 centre (0, 0) radius 35 projected
  point P0 (-0.006, -0.0789)
ref_plane "РабПлоскость1" through (-0.006, 0.0789, 30) normal (0, 0, 1) x (1, 0, 0)
